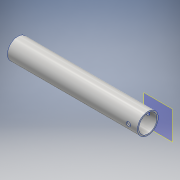
# Autodesk Inventor part: arm_back
Saved by Autodesk Inventor 2016 (Build 200138000, 138)
## iProperties
Created: 2016-09-22
Part Number: arm_back
Material: Aluminum 6061
Document SubType Name: Modeling
Designer: Jakub
Density: 2.7 g/cm^3
Appearance: Aluminum - Flat
Mass: 12.6802 g
Surface Area: 95.0684 cm^2
Volume: 4.69637 cm^3
Author: Jakub
Autodesk Inventor part; units mm, degrees
ref_plane "YZ Plane" through (0, 0, 0) normal (1, 0, 0) x (0, 1, 0)
ref_plane "XZ Plane" through (0, 0, 0) normal (0, 1, 0) x (-1, 0, 0)
ref_plane "XY Plane" through (0, 0, 0) normal (0, 0, 1) x (1, 0, 0)
sketch "Sketch1" plane through (0, 0, 0) normal (1, 0, 0) x (0, 1, 0)
  circle A0 centre (0, 0) radius 8
  circle A1 centre (0, 0) radius 7
  dimension "d0" = 16
  dimension "d1" = 14
  constraints: 2 centre point, 2 coincident
  measures "d0" diameter of A0
  measures "d1" diameter of A1
extrude "Extrusion1" add sketch "Sketch1" along normal blind 100
sketch "Sketch2" plane through (100, 0, 0) normal (1, 0, 0) x (0, 0, -1)
  circle A0 centre (0, 0) radius 8 projected
  line L0 (0, 8) -> (0, -8)
  constraints: 2 end point, 2 point on circle, 1 vertical
ref_plane "Work Plane1" through (100, 8, 0) normal (0, 1, 0) x (-1, 0, 0)
sketch "Sketch3" plane through (100, 8, 0) normal (0, 1, 0) x (-1, 0, 0)
  line L0 (0, 8) -> (0, -8) projected
  line L1 (0, 0) -> (7, 0)
  circle A0 centre (7, 0) radius 1.6
  point P0 (100, 0)
  dimension "d4" = 7
  dimension "d5" = 3.2
  constraints: 2 end point, 1 centre point, 1 coincident, 1 horizontal, 1 midpoint
  measures "d4" distance of L1.start L1.end
  measures "d5" diameter of A0
extrude "Extrusion2" cut sketch "Sketch3" against normal through all
body "Solid1"
